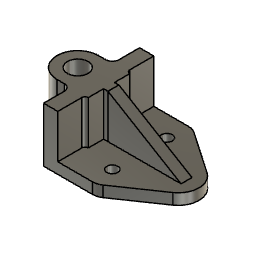
A3 (Autodesk Fusion 360 design; units mm, degrees)
Autodesk Fusion 360 part; units mm, degrees
sketch "Baza" plane through (0, 0, 0) normal (0, 0, 1) x (1, 0, 0)
  line L0 (16.2203, 44) -> (-15.5, 44)
  line L1 (-15.5, -22) -> (-15.5, -44)
  line L2 (-15.5, -44) -> (16.3266, -44)
  circle A0 centre (15.5, 25) radius 5
  circle A1 centre (15.5, -25) radius 5
  line L3 (15.5, 44) -> (51.5, 44) construction
  line L4 (15.5, -44) -> (51.5, -44) construction
  line L5 (51.5, 44) -> (51.5, -44) construction
  line L6 (-40, 0) -> (51.5, 0) construction
  line L7 (15.5, 25) -> (15.5, 20) construction
  line L8 (15.5, -20) -> (15.5, -25) construction
  line L9 (-15.5, 44) -> (-28.5, 44)
  line L10 (-28.5, 44) -> (-28.5, 25)
  line L11 (-28.5, -44) -> (-15.5, -44)
  line L12 (-12.5, -19) -> (-12.4999, -19) construction
  line L13 (-41.2176, -9.5) -> (-41.2176, 9.5) construction
  line L14 (-12.5, 19) -> (-12.4999, 19) construction
  circle A2 centre (-41.2176, 0) radius 9.5
  line L15 (-28.5, -25) -> (-28.5, -44)
  line L16 (-34.5, 19) -> (-41.2176, 19)
  arc A3 (-34.5, 19) -> (-28.5, 25) centre (-34.5, 25) ccw
  line L17 (-34.5, -19) -> (-41.2176, -19)
  arc A4 (-28.5, -25) -> (-34.5, -19) centre (-34.5, -25) ccw
  arc A5 (-41.2176, 19) -> (-41.2176, -19) centre (-41.2176, 0) ccw
  line L18 (-15.5, 44) -> (-15.5, 22)
  arc A6 (-15.5, 22) -> (-12.4999, 19) centre (-12.5, 22) ccw
  arc A7 (-12.4999, -19) -> (-15.5, -22) centre (-12.5, -22) ccw
  line L19 (-12.5, 4.9885) -> (-8.5, 4.9885)
  line L20 (-8.5, 4.9885) -> (-8.5, -5.0115)
  line L21 (-8.5, -5.0115) -> (-12.5, -5.0115)
  line L22 (-12.5, 19) -> (-12.5, 4.9885)
  line L23 (-12.5, -5.0115) -> (-12.5, -19)
  line L24 (64.6465, -13.1465) -> (64.935, -13.435) construction
  line L25 (51.5, 0) -> (70.5, 0) construction
  line L26 (64.6437, 13.1437) -> (64.935, 13.435) construction
  line L27 (61.6515, 15.6805) -> (23.5586, 41.7307)
  line L28 (61.6703, -15.6734) -> (23.6778, -41.7219)
  arc A8 (16.3266, -44) -> (23.6778, -41.7219) centre (16.3266, -31) ccw
  arc A9 (23.5586, 41.7307) -> (16.2203, 44) centre (16.2203, 31) ccw
  arc A10 (61.6703, -15.6734) -> (61.6515, 15.6805) centre (50.9262, -0.0029) ccw
  dimension "d1" = 88
  dimension "d2" = 31
  dimension "d3" = 50
  dimension "d5" = 10
  dimension "d6" = 10
  dimension "d7" = 36
  dimension "d12" = 13
  dimension "d13" = 38
  dimension "d15" = 3
  dimension "d16" = 19
  dimension "d18" = 6
  dimension "d20" = 6
  dimension "d21" = 3
  dimension "d22" = 3
  dimension "d23" = 10
  dimension "d24" = 20
  dimension "d27" = 13
  dimension "d28" = 13
  dimension "d29" = 19
  constraint horizontal L0
  constraint perpendicular L0 L1
  constraint parallel L0 L2
  constraint coincident A0.centre L7.start
  constraint coincident A1.centre L8.end
  constraint parallel L0 L3
  constraint perpendicular L4 L7
  constraint perpendicular L4 L5
  constraint midpoint L5 L6.end
  constraint perpendicular L5 L6
  constraint coincident A1 L8.start
  constraint collinear L7 L8
  constraint coincident A0 L7.end
  constraint horizontal L9
  constraint vertical L10
  constraint horizontal L11
  constraint vertical L22
  constraint vertical L13
  constraint concentric A2 A5
  constraint tangent L16 A5
  constraint coincident L11.start L10
  constraint tangent L16 A3
  constraint tangent L10 A3
  constraint tangent L17 A5
  constraint perpendicular L13 L17
  constraint coincident L9.end L15
  constraint tangent L15 A4
  constraint tangent L17 A4
  constraint coincident A2 L13.end
  constraint coincident L13 A2.centre
  constraint coincident A2 L13.start
  constraint perpendicular L2 L18
  constraint coincident L1.end L18
  constraint tangent L14 A6
  constraint tangent L18 A6
  constraint coincident L0.end L1
  constraint tangent L1 A7
  constraint tangent L12 A7
  constraint horizontal L19
  constraint vertical L20
  constraint horizontal L21
  constraint collinear L22 L23
  constraint horizontal L25
  constraint coincident L4.start L2
  constraint tangent L28 A8
  constraint tangent L2 A8
  constraint coincident L3.start L0
  constraint tangent L27 A9
  constraint tangent L0 A9
  constraint coincident L26.end L27
  constraint coincident L24.end L28
  constraint tangent L27 A10
  constraint tangent L28 A10
  constraint coincident A10 L26.start
  constraint coincident A10 L24.start
  measures "d1" distance of L0.end L1.end
  measures "d2" distance of L1.end L4.start
  measures "d3" distance of A0.centre A1.centre
  measures "d5" diameter of A0
  measures "d6" diameter of A1
  measures "d7" distance of L3.start L3.end
  measures "d12" distance of L0.end L9.end
  measures "d13" distance of L14.start L12.start
  measures "d15" distance of L1 L12.start
  measures "d16" diameter of A2
  measures "d18" radius of A3
  measures "d20" radius of A4
  measures "d21" radius of A6
  measures "d22" radius of A7
  measures "d23" distance of L19.end L20.end
  measures "d24" horizontal distance of L9.end L19.end
  measures "d27" radius of A8
  measures "d28" radius of A9
  measures "d29" radius of A10
extrude "Extrude1" add sketch "Baza" along normal blind 50 contours L1 L9 L10 L11 L15 L16 A3 L17 A4 A5 L18 A6 A7 L19 L20 L21 L22 L23
extrude "Extrude2" add sketch "Baza" along normal blind 10 contours L0 L1 L2 L18 A6 A7 L19 L20 L21 L22 L23 L27 L28 A8 A9 A10
sketch "Triunghi" plane through (0, 0, 0) normal (0, 1, 0) x (1, 0, 0)
  line L0 (-8.5, -50) -> (-8.5, -10)
  line L1 (-8.5, -10) -> (58.5, -10)
  line L2 (-15.5, 0) -> (16.3266, 0)
  line L3 (-15.5, -10) -> (-15.5, -50)
  line L4 (-8.5, -50) -> (58.5, -10)
  dimension "d34" = 10
  dimension "d41" = 40
  dimension "d42" = 67
  constraint vertical L0
  constraint perpendicular L0 L1
  measures "d34" distance of L1 L2
  measures "d41" distance of L0.start L0.end
  measures "d42" distance of L0.end L1.end
extrude "Extrude3" add sketch "Triunghi" along normal mid plane 10
named bodies: "A3"
